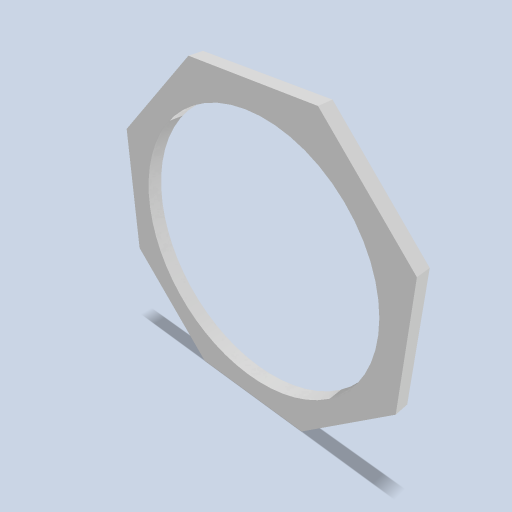
# Autodesk Inventor part: Bracket
Saved by Autodesk Inventor 2023 (Build 270158000, 158)
## iProperties
Created: 2022-10-10
Part Number: Bracket
Material: Generic
Document SubType Name: Modeling
Designer: Nathan
Density: 1 g/cm^3
Appearance: Default
Mass: 625.034 g
Surface Area: 1110.33 cm^2
Volume: 625.034 cm^3
Author: Nathan
Autodesk Inventor part; units mm, degrees
ref_plane "YZ Plane" through (0, 0, 0) normal (1, 0, 0) x (0, 1, 0)
ref_plane "XZ Plane" through (0, 0, 0) normal (0, 1, 0) x (-1, 0, 0)
ref_plane "XY Plane" through (0, 0, 0) normal (0, 0, 1) x (1, 0, 0)
sketch "Sketch1" plane through (0, 0, 0) normal (0, 0, 1) x (1, 0, 0)
  circle A0 centre (190.5, 190.5) radius 161.29
  circle A1 centre (190.5, 190.5) radius 161.29
  line L0 (190.5, 377.5583) -> (190.5, 351.79)
  line L1 (190.5, 3.4417) -> (190.5, 29.21)
  line L2 (0, 269.4113) -> (111.5887, 381)
  line L3 (0, 269.4113) -> (157.8102, 269.4113) construction
  line L4 (0, 111.5878) -> (111.5895, 0)
  line L5 (269.4113, 0) -> (381, 111.5903)
  line L6 (380.9968, 269.4113) -> (269.4113, 381)
  line L7 (0, 0) -> (380.9968, 0)
  line L8 (380.9968, 0) -> (380.9968, 380.9968)
  line L9 (380.9968, 380.9968) -> (0, 380.9968)
  line L10 (0, 380.9968) -> (0, 0)
  point P0 (111.5855, 380.9968)
  point P1 (111.5895, 0)
  point P2 (380.9968, 111.5871)
  point P3 (269.4145, 380.9968)
  dimension "d3" = 322.58
  dimension "d25" = 25.7683
  dimension "d26" = 25.7683
  dimension "d27" = 45
  dimension "d28" = 157.8102
  dimension "d30" = 157.8235
  dimension "d32" = 157.8218
  dimension "d40" = 157.808
  dimension "d42" = 380.9968
  dimension "d43" = 380.9968
  dimension "d44" = 190.5
  dimension "d45" = 190.5
  dimension "d46" = 111.5878
  constraints: 22 end point, 2 centre point, 2 horizontal, 2 parallel, 2 perpendicular, 2 point on circle, 2 vertical, 1 coincident, 1 concentric, 1 equal length
  measures "d3" diameter of A0
  measures "d25" distance of L0.start L0.end
  measures "d26" distance of L1.start L1.end
  measures "d27" angle of L3 L2
  measures "d28" distance of L2.start L2.end
  measures "d30" distance of L4.start L2.start
  measures "d32" distance of L5.start L4.end
  measures "d40" distance of L6.start L6.end
  measures "d42" distance of L8.end L9.end
  measures "d43" distance of L7.end L8.end
  measures "d44" horizontal distance of L7.start A1.centre
  measures "d45" horizontal distance of L7.start A0.centre
  measures "d46" vertical distance of L4.start L4.end
extrude "Extrusion2" add sketch "Sketch1" along normal blind 17.8562 contours L2 L9 L6 L8 L5 L7 L4 L10
body "Solid2"
